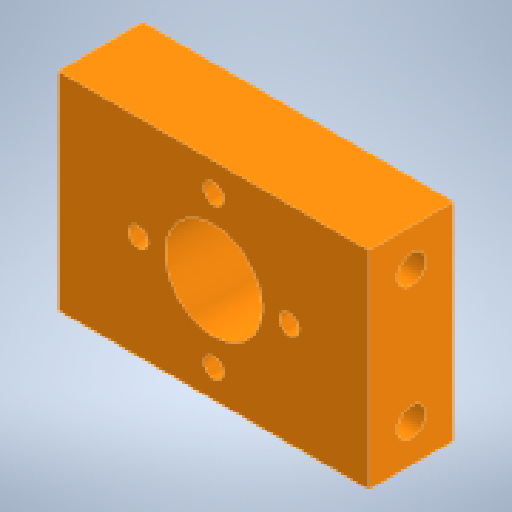
# Autodesk Inventor part: rosca_trapezoidal_001
Saved by Autodesk Inventor 2026 (Build 300175000, 175)
## iProperties
Created: 2025-11-26
Part Number: rosca_trapezoidal_001
Material: ABS Plastic
Document SubType Name: Modeling
Designer: Carlos Dias
Density: 1.06 g/cm^3
Appearance: Orange
Author: Carlos Dias
Autodesk Inventor part; units mm, degrees
ref_plane "YZ Plane" through (0, 0, 0) normal (1, 0, 0) x (0, 1, 0)
ref_plane "XZ Plane" through (0, 0, 0) normal (0, 1, 0) x (-1, 0, 0)
ref_plane "XY Plane" through (0, 0, 0) normal (0, 0, 1) x (1, 0, 0)
sketch "Sketch1" plane through (0, 0, 0) normal (0, 0, 1) x (1, 0, 0)
  line L0 (-16.5, 11) -> (16.5, 11)
  line L1 (16.5, 11) -> (16.5, -11)
  line L2 (16.5, -11) -> (-16.5, -11)
  line L3 (-16.5, -11) -> (-16.5, 11)
  line L4 (-16.5, 11) -> (16.5, -11) construction
  line L5 (16.5, 11) -> (-16.5, -11) construction
  line L6 (-16.5, 11) -> (16.5, -11) construction
  line L7 (16.5, 11) -> (-16.5, -11) construction
  circle A0 centre (0, 0) radius 5.15
  circle A1 centre (0, 8) radius 1.05
  circle A2 centre (-8, 0) radius 1.05
  circle A3 centre (0, -8) radius 1.05
  circle A4 centre (8, 0) radius 1.05
  dimension "d0" = 33
  dimension "d1" = 22
  dimension "d5" = 22
  dimension "d6" = 10.3
  dimension "d7" = 8
  dimension "d8" = 360
  dimension "d9" = 2.1
  constraints: 16 end point, 5 centre point, 4 coincident, 4 midpoint, 2 parallel, 1 horizontal, 1 perpendicular, 1 vertical alignment, 9 other
  measures "d0" distance of L0.start L0.end
  measures "d1" distance of L0.end L1.end
  measures "d5" distance of L7.end L6.start
  measures "d6" diameter of A0
  measures "d7" distance of point (0, 0) A1.centre
  measures "d9" diameter of A1
extrude "Extrusion1" add sketch "Sketch1" along normal mid plane 9
sketch "Sketch2" plane through (16.5, -11, 4.5) normal (1, 0, 0) x (0, 0, -1)
  circle A0 centre (4.5, 4) radius 1.5
  circle A1 centre (4.5, 18) radius 1.5
  line L0 (9, 0) -> (0, 0) projected
  line L1 (0, 11) -> (9, 11) construction
  line L2 (9, 22) -> (9, 0) projected
  line L3 (0, 0) -> (0, 22) projected
  point P0 (4.5, 11)
  point P1 (4.5, 0)
  dimension "d12" = 3
  dimension "d13" = 4
  constraints: 3 midpoint, 2 centre point, 2 end point, 2 vertical alignment, 1 equal radius, 1 horizontal, 1 other
  measures "d12" diameter of A1
  measures "d13" distance from line of L0 A0.centre
extrude "Extrusion2" cut sketch "Sketch2" against normal blind 5
body "Solid1"
